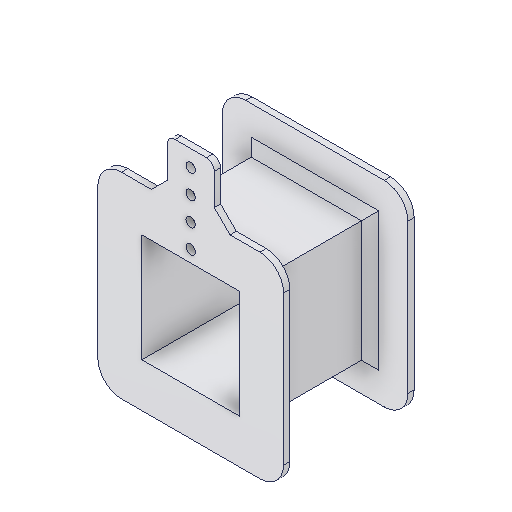
# Autodesk Inventor part: 3DP_ABS_Electromagnet_Coil_Holder
Saved by Autodesk Inventor 2025 (Build 290162010, 162A)
## iProperties
Created: 2018-05-26
Part Number: 3DP_ABS_Electromagnet_Coil_Holder
Material: ABS Plastic
Document SubType Name: Modeling
Designer: Andrzej
Density: 1.06 g/cm^3
Appearance: PTFE
Author: Andrzej
Autodesk Inventor part; units mm, degrees
ref_plane "YZ Plane" through (0, 0, 0) normal (1, 0, 0) x (0, 1, 0)
ref_plane "XZ Plane" through (0, 0, 0) normal (0, 1, 0) x (-1, 0, 0)
ref_plane "XY Plane" through (0, 0, 0) normal (0, 0, 1) x (1, 0, 0)
sketch "Sketch1" plane through (0, 0, 0) normal (0, 0, 1) x (1, 0, 0)
  line L0 (-6.2, 6.875) -> (6.2, 6.875)
  line L1 (6.2, 6.875) -> (6.2, -6.875)
  line L2 (6.2, -6.875) -> (-6.2, -6.875)
  line L3 (-6.2, -6.875) -> (-6.2, 6.875)
  line L4 (8.8, 12.475) -> (-8.8, 12.475)
  line L5 (-11.8, 9.475) -> (-11.8, -9.475)
  line L6 (-8.8, -12.475) -> (8.8, -12.475)
  line L7 (11.8, -9.475) -> (11.8, 9.475)
  arc A0 (-8.8, 12.475) -> (-11.8, 9.475) centre (-8.8, 9.475) ccw
  arc A1 (11.8, 9.475) -> (8.8, 12.475) centre (8.8, 9.475) ccw
  arc A2 (8.8, -12.475) -> (11.8, -9.475) centre (8.8, -9.475) ccw
  arc A3 (-11.8, -9.475) -> (-8.8, -12.475) centre (-8.8, -9.475) ccw
  point P0 (0, 0)
  dimension "d0" = 12.4
  dimension "d1" = 13.75
  dimension "d2" = 5.6
  dimension "d3" = 3
  dimension "d4" = 6.875
  dimension "d5" = 6.2
  dimension "d16" = 23.6
  dimension "d17" = 24.95
  constraints: 16 end point, 8 point on circle, 8 tangent, 4 centre point, 4 parallel, 3 equal radius, 2 perpendicular, 1 horizontal, 3 other
  measures "d0" distance of L1.end L2.end
  measures "d1" distance of L0.end L1.end
  measures "d2" distance between parallel lines of L0 L4
  measures "d3" radius of A0
  measures "d4" distance from line of point (0, 0) L0
  measures "d5" distance from line of L3 point (0, 0)
  measures "d16" distance between parallel lines of L7 L5
  measures "d17" distance between parallel lines of L6 L4
extrude "Extrusion1" add sketch "Sketch1" along normal blind 0.8
sketch "Sketch3" plane through (0, 0, 0) normal (0, 0, -1) x (-1, 0, 0)
  line L0 (-6.2, -6.875) -> (-6.2, 6.875) projected
  line L1 (-6.2, 6.875) -> (6.2, 6.875) projected
  line L2 (6.2, 6.875) -> (6.2, -6.875) projected
  line L3 (6.2, -6.875) -> (-6.2, -6.875) projected
  line L4 (8.8, 12.475) -> (-8.8, 12.475) projected
  arc A0 (-8.8, 12.475) -> (-11.8, 9.475) centre (-8.8, 9.475) ccw projected
  line L5 (-11.8, 9.475) -> (-11.8, -9.475) projected
  arc A1 (-11.8, -9.475) -> (-8.8, -12.475) centre (-8.8, -9.475) ccw projected
  line L6 (-8.8, -12.475) -> (8.8, -12.475) projected
  arc A2 (8.8, -12.475) -> (11.8, -9.475) centre (8.8, -9.475) ccw projected
  line L7 (11.8, -9.475) -> (11.8, 9.475) projected
  arc A3 (11.8, 9.475) -> (8.8, 12.475) centre (8.8, 9.475) ccw projected
  line L8 (7, -7.675) -> (7, 7.675)
  line L9 (7, 7.675) -> (-7, 7.675)
  line L10 (-7, 7.675) -> (-7, -7.675)
  line L11 (-7, -7.675) -> (7, -7.675)
  point P0 (0, 0)
  dimension "d11" = 0.8
  constraints: 8 end point, 3 other
  measures "d11" distance between parallel lines of L2 L8
extrude "Extrusion2" add sketch "Sketch3" along normal blind 15 contours L11 L10 L9 L8
sketch "Sketch4" plane through (0, 0, -15) normal (0, 0, -1) x (-1, 0, 0)
  line L0 (7, -7.675) -> (-7, -7.675) projected
  line L1 (-7, -7.675) -> (-7, 7.675) projected
  line L2 (-7, 7.675) -> (7, 7.675) projected
  line L3 (7, 7.675) -> (7, -7.675) projected
  line L4 (8.8, 12.475) -> (-8.8, 12.475) projected
  arc A0 (-8.8, 12.475) -> (-11.8, 9.475) centre (-8.8, 9.475) ccw projected
  line L5 (-11.8, 9.475) -> (-11.8, -9.475) projected
  arc A1 (-11.8, -9.475) -> (-8.8, -12.475) centre (-8.8, -9.475) ccw projected
  line L6 (-8.8, -12.475) -> (8.8, -12.475) projected
  arc A2 (8.8, -12.475) -> (11.8, -9.475) centre (8.8, -9.475) ccw projected
  line L7 (11.8, -9.475) -> (11.8, 9.475) projected
  arc A3 (11.8, 9.475) -> (8.8, 12.475) centre (8.8, 9.475) ccw projected
  line L8 (-6.2, 6.875) -> (6.2, 6.875) projected
  line L9 (6.2, 6.875) -> (6.2, -6.875) projected
  line L10 (6.2, -6.875) -> (-6.2, -6.875) projected
  line L11 (-6.2, -6.875) -> (-6.2, 6.875) projected
  line L12 (7, -7.675) -> (7, 7.675) projected
  line L13 (7, 7.675) -> (-7, 7.675) projected
  line L14 (-7, 7.675) -> (-7, -7.675) projected
  line L15 (-7, -7.675) -> (7, -7.675) projected
  point P0 (0, 0)
extrude "Extrusion3" add sketch "Sketch4" along normal blind 0.8 contours L0 L1 L2 L3 | A3 L7 A2 L6 A1 L5 A0 L4
chamfer "Chamfer1" distance 1.1 angle 45 8 edges at (7, 0, 0) (0, -7.675, 0) (0, 7.675, 0) (-7, 0, 0) (-7, 0, -15) (0, 7.675, -15) (0, -7.675, -15) (7, 0, -15)
sketch "Sketch5" plane through (0, 0, 0.8) normal (0, 0, 1) x (1, 0, 0)
  circle A0 centre (0, 8.375) radius 0.6
  line L0 (-6.2, 6.875) -> (6.2, 6.875) projected
  line L1 (11.8, -9.475) -> (11.8, 9.475) projected
  line L2 (-11.8, 9.475) -> (-11.8, -9.475) projected
  line L3 (6.2, 6.875) -> (6.2, -6.875) projected
  line L4 (6.2, -6.875) -> (-6.2, -6.875) projected
  line L5 (-6.2, -6.875) -> (-6.2, 6.875) projected
  line L6 (-6.2, 6.875) -> (6.2, 6.875) projected
  line L7 (8.8, 12.475) -> (-8.8, 12.475) projected
  arc A1 (-8.8, 12.475) -> (-11.8, 9.475) centre (-8.8, 9.475) ccw projected
  line L8 (-11.8, 9.475) -> (-11.8, -9.475) projected
  arc A2 (-11.8, -9.475) -> (-8.8, -12.475) centre (-8.8, -9.475) ccw projected
  line L9 (-8.8, -12.475) -> (8.8, -12.475) projected
  arc A3 (8.8, -12.475) -> (11.8, -9.475) centre (8.8, -9.475) ccw projected
  line L10 (11.8, -9.475) -> (11.8, 9.475) projected
  arc A4 (11.8, 9.475) -> (8.8, 12.475) centre (8.8, 9.475) ccw projected
  line L11 (-8.8, 12.475) -> (8.8, 12.475) projected
  line L12 (3, 12.475) -> (-3, 12.475)
  line L13 (-3, 12.475) -> (-3, 19.475)
  line L14 (-3, 19.475) -> (3, 19.475)
  line L15 (3, 19.475) -> (3, 12.475)
  circle A5 centre (0, 11.375) radius 0.6
  circle A6 centre (0, 14.375) radius 0.6
  circle A7 centre (0, 17.375) radius 0.6
  point P0 (0, 0)
  dimension "d21" = 1.2
  dimension "d22" = 1.5
  dimension "d23" = 11.8
  dimension "d24" = 23.6
  dimension "d27" = 6
  dimension "d28" = 7
  dimension "d29" = 8.8
  dimension "d32" = 3
  constraints: 8 end point, 4 centre point, 2 parallel, 1 horizontal, 1 perpendicular, 1 point on line, 1 vertical, 6 other
  measures "d21" diameter of A0
  measures "d22" distance from line of L0 A0.centre
  measures "d23" distance from line of L1 A0.centre
  measures "d24" distance between parallel lines of L2 L1
  measures "d27" distance of L13.end L14.end
  measures "d28" distance of L12.end L13.end
  measures "d29" distance between parallel lines of L15 L10
  measures "d32" distance of A0.centre A5.centre
extrude "Extrusion4" add sketch "Sketch5" against normal up to surface (0.8 mm away) contours L7 L13 L14 L15
chamfer "Chamfer2" distance 2 angle 45 2 edges at (-3, 12.475, 0.4) (3, 12.475, 0.4)
extrude "Extrusion5" cut sketch "Sketch5" against normal blind 10 contours A0 | A5
fillet "Fillet1" radius 1 2 edges at (-3, 19.475, 0.4) (3, 19.475, 0.4)
equation "\"d4\" = 0.5 * d1"
equation "\"d5\" = 0.5 * d0"
equation "\"d23\" = 0.5 * d24"
equation "\"d29\" = -0.5 * d27 + 0.5 * d24"
body "Solid1"
